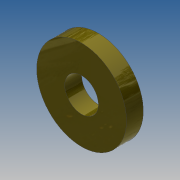
# Autodesk Inventor part: Dichtrign_ra8846s
Saved by Autodesk Inventor 2021 (Build 250183000, 183)
## iProperties
Created: 2020-12-18
Part Number: Dichtrign_ra8846s
Material: PC/ABS-Kunststoff
Document SubType Name: Modeling
Designer: Sander
Density: 0.357273 g/cm^3
Appearance: Glatt - Weiß
Mass: 0.0231496 g
Surface Area: 1.3823 cm^2
Volume: 0.0647953 cm^3
Author: Sander
Autodesk Inventor part; units mm, degrees
ref_plane "YZ-Ebene" through (0, 0, 0) normal (1, 0, 0) x (0, 1, 0)
ref_plane "XZ-Ebene" through (0, 0, 0) normal (0, 1, 0) x (-1, 0, 0)
ref_plane "XY-Ebene" through (0, 0, 0) normal (0, 0, 1) x (1, 0, 0)
sketch "Skizze1" plane through (0, 0, 0) normal (0, 0, 1) x (1, 0, 0)
  line L0 (-4.8, 0) -> (0.8, 0) projected
  line L1 (0, -0.3) -> (0, 1.8) projected
  line L2 (-4, 1.5) -> (-1.5, 1.5)
  line L3 (-1.5, 1.5) -> (-1.5, 0)
  line L4 (-1.5, 0) -> (-4, 0)
  line L5 (-4, 0) -> (-4, 1.5)
  point P0 (0, 0)
  dimension "d0" = 1.5
  dimension "d1" = 1.5
  dimension "d2" = 4
  constraints: 8 end point, 2 parallel, 1 horizontal, 1 perpendicular, 1 point on line
  measures "d0" distance of L4.end L2.start
  measures "d1" distance of point (0, 0) L3.end
  measures "d2" distance of point (0, 0) L4.end
revolve "Umdrehung1" add sketch "Skizze1" angle 360 about axis through (0, -10, 0) along (0, 1, 0)
